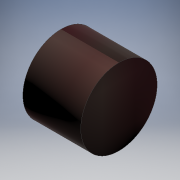
# Autodesk Inventor part: rond
Saved by Autodesk Inventor 2017 (Build 210142000, 142)
## iProperties
Created: 2018-11-10
Part Number: rond
Material: Generic
Document SubType Name: Modeling
Designer: Antoine Blaud
Density: 1 g/cm^3
Appearance: Default
Author: Antoine Blaud
Autodesk Inventor part; units mm, degrees
ref_plane "YZ Plane" through (0, 0, 0) normal (1, 0, 0) x (0, 1, 0)
ref_plane "XZ Plane" through (0, 0, 0) normal (0, 1, 0) x (-1, 0, 0)
ref_plane "XY Plane" through (0, 0, 0) normal (0, 0, 1) x (1, 0, 0)
sketch "Sketch1" plane through (0, 0, 0) normal (1, 0, 0) x (0, 1, 0)
  circle A0 centre (0, 0) radius 4.191
  circle A1 centre (0, 0) radius 3.81
  dimension "d0" = 8.382
  dimension "d1" = 7.62
  constraints: 2 centre point, 2 coincident
  measures "d0" diameter of A0
  measures "d1" diameter of A1
extrude "Extrusion1" add sketch "Sketch1" along normal blind 1.27
sketch "Sketch2" plane through (0, 0, 0) normal (-1, 0, 0) x (0, 0, 1)
  circle A0 centre (0, 0) radius 4.191
  circle A1 centre (0, 0) radius 3.81
  dimension "d5" = 8.382
  dimension "d4" = 7.62
  constraints: 2 centre point, 2 coincident
  measures "d5" diameter of A0
  measures "d4" diameter of A1
extrude "Extrusion2" add sketch "Sketch2" along normal blind 1.27
sketch "Sketch3" plane through (-1.27, 0, 0) normal (-1, 0, 0) x (0, 0, 1)
  circle A0 centre (0, 0) radius 4.191
  circle A1 centre (0, 0) radius 3.81
  dimension "d10" = 8.382
  dimension "d9" = 7.62
  constraints: 2 centre point, 2 coincident
  measures "d10" diameter of A0
  measures "d9" diameter of A1
extrude "Extrusion3" add sketch "Sketch3" along normal blind 1.27
sketch "Sketch4" plane through (1.27, 0, 0) normal (1, 0, 0) x (0, 0, -1)
  circle A0 centre (0, 0) radius 4.191
  circle A1 centre (0, 0) radius 3.81
  dimension "d15" = 8.382
  dimension "d14" = 7.62
  constraints: 2 centre point, 2 coincident
  measures "d15" diameter of A0
  measures "d14" diameter of A1
extrude "Extrusion4" add sketch "Sketch4" along normal blind 1.27
sketch "Sketch5" plane through (2.54, 0, 0) normal (1, 0, 0) x (0, 0, -1)
  circle A0 centre (0, 0) radius 4.191
  circle A1 centre (0, 0) radius 3.81
  dimension "d20" = 8.382
  dimension "d19" = 7.62
  constraints: 2 centre point, 2 coincident
  measures "d20" diameter of A0
  measures "d19" diameter of A1
extrude "Extrusion5" add sketch "Sketch5" along normal blind 1.27
sketch "Sketch6" plane through (3.81, 0, 0) normal (1, 0, 0) x (0, 0, -1)
  circle A0 centre (0, 0) radius 3.81
  constraints: 1 centre point, 1 coincident
extrude "Extrusion6" add sketch "Sketch6" against normal blind 0.508
body "Solid1"
